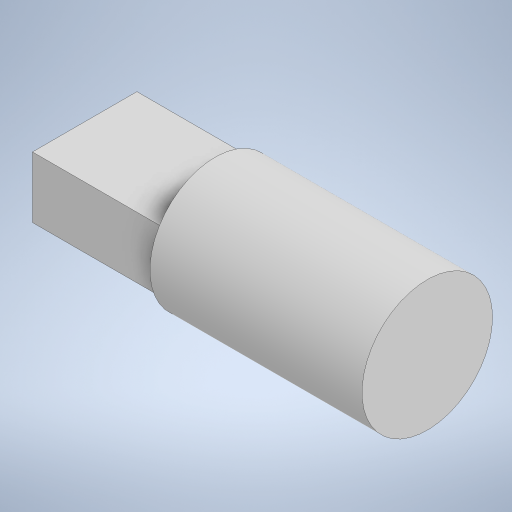
# Autodesk Inventor part: Part6 x 2
Saved by Autodesk Inventor 2023.1 (Build 271208000, 208)
## iProperties
Created: 2022-10-25
Part Number: Part6 x 2
Material: Generic
Document SubType Name: Modeling
Designer: jshin23
Density: 1 g/cm^3
Appearance: Default
Author: jshin23
Autodesk Inventor part; units mm, degrees
ref_plane "YZ Plane" through (0, 0, 0) normal (1, 0, 0) x (0, 1, 0)
ref_plane "XZ Plane" through (0, 0, 0) normal (0, 1, 0) x (-1, 0, 0)
ref_plane "XY Plane" through (0, 0, 0) normal (0, 0, 1) x (1, 0, 0)
sketch "Sketch1" plane through (0, 0, 0) normal (0, 1, 0) x (-1, 0, 0)
  line L0 (0, 0) -> (20.32, 0)
  line L1 (20.32, 0) -> (20.32, -16.256)
  line L2 (20.32, -16.256) -> (0, -16.256)
  line L3 (0, -16.256) -> (0, 0)
  dimension "d0" = 20.32
  dimension "d1" = 16.256
  constraints: 8 end point, 2 parallel, 1 horizontal, 1 perpendicular
  measures "d0" distance of L1.end L2.end
  measures "d1" distance of L0.end L1.end
extrude "Extrusion1" add sketch "Sketch1" along normal blind 9.525
sketch "Sketch2" plane through (0, 0, 0) normal (1, 0, 0) x (0, 0, -1)
  circle A0 centre (8.128, 4.7625) radius 10.16
  line L0 (0, 9.525) -> (16.256, 9.525) projected
  line L1 (0, 0) -> (0, 9.525) projected
  line L2 (16.256, 0) -> (0, 0) projected
  line L3 (0, 0) -> (0, 9.525) projected
  point P0 (8.128, 0)
  point P1 (0, 4.7625)
  dimension "d4" = 20.32
  dimension "d9" = 0
  dimension "d10" = 0
  constraints: 2 midpoint, 1 centre point
  measures "d4" diameter of A0
  measures "d9" horizontal distance of A0.centre point (8.128, 0)
  measures "d10" vertical distance of A0.centre point (0, 4.763)
extrude "Extrusion2" add sketch "Sketch2" along normal blind 33.02
scale "Scale1" factors (0.98, 0.98, 0.98) then translate (0.3302, 0.0953, -0.1626) bodies 1
body "Solid1"
